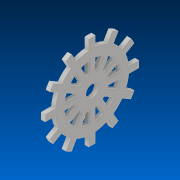
# Autodesk Inventor part: paddlewheel_inner
Saved by Autodesk Inventor 2019 (Build 230136000, 136)
## iProperties
Created: 2018-08-23
Part Number: paddlewheel_inner
Material: Generic
Document SubType Name: Modeling
Designer: Kitte_X
Density: 1 g/cm^3
Appearance: Default
Author: Kitte_X
Autodesk Inventor part; units mm, degrees
ref_plane "YZ Plane" through (0, 0, 0) normal (1, 0, 0) x (0, 1, 0)
ref_plane "XZ Plane" through (0, 0, 0) normal (0, 1, 0) x (-1, 0, 0)
ref_plane "XY Plane" through (0, 0, 0) normal (0, 0, 1) x (1, 0, 0)
sketch "Sketch1" plane through (0, 0, 0) normal (1, 0, 0) x (0, 1, 0)
  circle A0 centre (0, 0) radius 10
  line L0 (5.4386, -55.161) -> (-5.4386, -55.161) construction
  line L1 (-5.4386, -76.0008) -> (-5.4386, -59.753)
  line L2 (-5, -44.8834) -> (-5, -25.7185)
  line L3 (5, -25.7185) -> (5, -44.8834)
  line L4 (5.4386, -59.753) -> (5.4386, -76.0008)
  arc A1 (-5.4386, -76.0008) -> (5.4386, -76.0008) centre (0, 0) ccw
  line L5 (18.1116, -41.3702) -> (8.5291, -24.7729)
  line L6 (17.1894, -19.7729) -> (26.7718, -36.3702)
  line L7 (34.5865, -49.0283) -> (42.7104, -63.0993)
  arc A2 (33.2904, -68.5379) -> (42.7104, -63.0993) centre (0, 0) ccw
  line L8 (33.2904, -68.5379) -> (25.1665, -54.4669)
  line L9 (36.3702, -26.7718) -> (19.7729, -17.1894)
  line L10 (24.7729, -8.5291) -> (41.3702, -18.1116)
  line L11 (54.4669, -25.1665) -> (68.5379, -33.2904)
  arc A3 (63.0993, -42.7104) -> (68.5379, -33.2904) centre (0, 0) ccw
  line L12 (63.0993, -42.7104) -> (49.0283, -34.5865)
  line L13 (44.8834, -5) -> (25.7185, -5)
  line L14 (25.7185, 5) -> (44.8834, 5)
  line L15 (59.753, 5.4386) -> (76.0008, 5.4386)
  arc A4 (76.0008, -5.4386) -> (76.0008, 5.4386) centre (0, 0) ccw
  line L16 (76.0008, -5.4386) -> (59.753, -5.4386)
  line L17 (41.3702, 18.1116) -> (24.7729, 8.5291)
  line L18 (19.7729, 17.1894) -> (36.3702, 26.7718)
  line L19 (49.0283, 34.5865) -> (63.0993, 42.7104)
  arc A5 (68.5379, 33.2904) -> (63.0993, 42.7104) centre (0, 0) ccw
  line L20 (68.5379, 33.2904) -> (54.4669, 25.1665)
  line L21 (26.7718, 36.3702) -> (17.1894, 19.7729)
  line L22 (8.5291, 24.7729) -> (18.1116, 41.3702)
  line L23 (25.1665, 54.4669) -> (33.2904, 68.5379)
  arc A6 (42.7104, 63.0993) -> (33.2904, 68.5379) centre (0, 0) ccw
  line L24 (42.7104, 63.0993) -> (34.5865, 49.0283)
  line L25 (5, 44.8834) -> (5, 25.7185)
  line L26 (-5, 25.7185) -> (-5, 44.8834)
  line L27 (-5.4386, 59.753) -> (-5.4386, 76.0008)
  arc A7 (5.4386, 76.0008) -> (-5.4386, 76.0008) centre (0, 0) ccw
  line L28 (5.4386, 76.0008) -> (5.4386, 59.753)
  line L29 (-18.1116, 41.3702) -> (-8.5291, 24.7729)
  line L30 (-17.1894, 19.7729) -> (-26.7718, 36.3702)
  line L31 (-34.5865, 49.0283) -> (-42.7104, 63.0993)
  arc A8 (-33.2904, 68.5379) -> (-42.7104, 63.0993) centre (0, 0) ccw
  line L32 (-33.2904, 68.5379) -> (-25.1665, 54.4669)
  line L33 (-36.3702, 26.7718) -> (-19.7729, 17.1894)
  line L34 (-24.7729, 8.5291) -> (-41.3702, 18.1116)
  line L35 (-54.4669, 25.1665) -> (-68.5379, 33.2904)
  arc A9 (-63.0993, 42.7104) -> (-68.5379, 33.2904) centre (0, 0) ccw
  line L36 (-63.0993, 42.7104) -> (-49.0283, 34.5865)
  line L37 (-44.8834, 5) -> (-25.7185, 5)
  line L38 (-25.7185, -5) -> (-44.8834, -5)
  line L39 (-59.753, -5.4386) -> (-76.0008, -5.4386)
  arc A10 (-76.0008, 5.4386) -> (-76.0008, -5.4386) centre (0, 0) ccw
  line L40 (-76.0008, 5.4386) -> (-59.753, 5.4386)
  line L41 (-41.3702, -18.1116) -> (-24.7729, -8.5291)
  line L42 (-19.7729, -17.1894) -> (-36.3702, -26.7718)
  line L43 (-49.0283, -34.5865) -> (-63.0993, -42.7104)
  arc A11 (-68.5379, -33.2904) -> (-63.0993, -42.7104) centre (0, 0) ccw
  line L44 (-68.5379, -33.2904) -> (-54.4669, -25.1665)
  line L45 (-26.7718, -36.3702) -> (-17.1894, -19.7729)
  line L46 (-8.5291, -24.7729) -> (-18.1116, -41.3702)
  line L47 (-25.1665, -54.4669) -> (-33.2904, -68.5379)
  arc A12 (-42.7104, -63.0993) -> (-33.2904, -68.5379) centre (0, 0) ccw
  line L48 (-42.7104, -63.0993) -> (-34.5865, -49.0283)
  arc A13 (5, -44.8834) -> (18.1116, -41.3702) centre (0, 0) ccw
  arc A14 (-18.1116, -41.3702) -> (-5, -44.8834) centre (0, 0) ccw
  arc A15 (-36.3702, -26.7718) -> (-26.7718, -36.3702) centre (0, 0) ccw
  arc A16 (-44.8834, -5) -> (-41.3702, -18.1116) centre (0, 0) ccw
  arc A17 (-24.7729, 8.5291) -> (-25.7185, 5) centre (0, 0) ccw
  arc A18 (-41.3702, 18.1116) -> (-44.8834, 5) centre (0, 0) ccw
  arc A19 (-26.7718, 36.3702) -> (-36.3702, 26.7718) centre (0, 0) ccw
  arc A20 (-17.1894, 19.7729) -> (-19.7729, 17.1894) centre (0, 0) ccw
  arc A21 (-5, 44.8834) -> (-18.1116, 41.3702) centre (0, 0) ccw
  arc A22 (-5, 25.7185) -> (-8.5291, 24.7729) centre (0, 0) ccw
  arc A23 (8.5291, 24.7729) -> (5, 25.7185) centre (0, 0) ccw
  arc A24 (18.1116, 41.3702) -> (5, 44.8834) centre (0, 0) ccw
  arc A25 (36.3702, 26.7718) -> (26.7718, 36.3702) centre (0, 0) ccw
  arc A26 (19.7729, 17.1894) -> (17.1894, 19.7729) centre (0, 0) ccw
  arc A27 (25.7185, 5) -> (24.7729, 8.5291) centre (0, 0) ccw
  arc A28 (26.7718, -36.3702) -> (36.3702, -26.7718) centre (0, 0) ccw
  arc A29 (24.7729, -8.5291) -> (25.7185, -5) centre (0, 0) ccw
  arc A30 (17.1894, -19.7729) -> (19.7729, -17.1894) centre (0, 0) ccw
  arc A31 (5, -25.7185) -> (8.5291, -24.7729) centre (0, 0) ccw
  arc A32 (-8.5291, -24.7729) -> (-5, -25.7185) centre (0, 0) ccw
  arc A33 (-25.7185, -5) -> (-24.7729, -8.5291) centre (0, 0) ccw
  arc A34 (-19.7729, -17.1894) -> (-17.1894, -19.7729) centre (0, 0) ccw
  arc A35 (41.3702, -18.1116) -> (44.8834, -5) centre (0, 0) ccw
  arc A36 (44.8834, 5) -> (41.3702, 18.1116) centre (0, 0) ccw
  arc A37 (-49.0283, -34.5865) -> (-34.5865, -49.0283) centre (0, 0) ccw
  arc A38 (-25.1665, -54.4669) -> (-5.4386, -59.753) centre (0, 0) ccw
  arc A39 (5.4386, -59.753) -> (25.1665, -54.4669) centre (0, 0) ccw
  arc A40 (34.5865, -49.0283) -> (49.0283, -34.5865) centre (0, 0) ccw
  arc A41 (54.4669, -25.1665) -> (59.753, -5.4386) centre (0, 0) ccw
  arc A42 (59.753, 5.4386) -> (54.4669, 25.1665) centre (0, 0) ccw
  arc A43 (49.0283, 34.5865) -> (34.5865, 49.0283) centre (0, 0) ccw
  arc A44 (25.1665, 54.4669) -> (5.4386, 59.753) centre (0, 0) ccw
  arc A45 (-5.4386, 59.753) -> (-25.1665, 54.4669) centre (0, 0) ccw
  arc A46 (-34.5865, 49.0283) -> (-49.0283, 34.5865) centre (0, 0) ccw
  arc A47 (-54.4669, 25.1665) -> (-59.753, 5.4386) centre (0, 0) ccw
  arc A48 (-59.753, -5.4386) -> (-54.4669, -25.1665) centre (0, 0) ccw
  point P0 (0, -55.161)
  point P1 (32.2905, -45.0516)
  point P2 (22.8705, -50.4902)
  point P3 (50.4902, -22.8705)
  point P4 (45.0516, -32.2905)
  point P5 (55.161, 5.4386)
  point P6 (55.161, -5.4386)
  point P7 (45.0516, 32.2905)
  point P8 (50.4902, 22.8705)
  point P9 (22.8705, 50.4902)
  point P10 (32.2905, 45.0516)
  point P11 (-5.4386, 55.161)
  point P12 (5.4386, 55.161)
  point P13 (-32.2905, 45.0516)
  point P14 (-22.8705, 50.4902)
  point P15 (-50.4902, 22.8705)
  point P16 (-45.0516, 32.2905)
  point P17 (-55.161, -5.4386)
  point P18 (-55.161, 5.4386)
  point P19 (-45.0516, -32.2905)
  point P20 (-50.4902, -22.8705)
  point P21 (-22.8705, -50.4902)
  point P22 (-32.2905, -45.0516)
  dimension "d0" = 20
  dimension "d19" = 360
  constraints: 98 end point, 96 point on circle, 49 centre point, 24 point on line, 4 parallel, 3 coincident, 2 midpoint, 2 perpendicular, 2 vertical, 1 vertical alignment, 193 other
  measures "d0" diameter of A0
extrude "Extrusion2" add sketch "Sketch1" along normal blind 6.35
body "Solid2"
